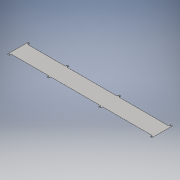
# Autodesk Inventor part: Baseplate
Saved by Autodesk Inventor 2016 (Build 200138000, 138)
## iProperties
Created: 2017-06-28
Part Number: Baseplate
Material: Generic
Document SubType Name: Modeling
Designer: Roeder
Density: 1 g/cm^3
Appearance: Default
Author: Roeder
Autodesk Inventor part; units mm, degrees
ref_plane "YZ Plane" through (0, 0, 0) normal (1, 0, 0) x (0, 1, 0)
ref_plane "XZ Plane" through (0, 0, 0) normal (0, 1, 0) x (-1, 0, 0)
ref_plane "XY Plane" through (0, 0, 0) normal (0, 0, 1) x (1, 0, 0)
sketch "Sketch1" plane through (0, 0, 0) normal (0, 0, 1) x (1, 0, 0)
  line L0 (-836.3865, 0) -> (4049.6135, 0) projected
  line L1 (0, -497.7012) -> (0, 202.2988) projected
  line L2 (-93.3865, 52.2988) -> (3306.6135, 52.2988)
  line L3 (3306.6135, 52.2988) -> (3306.6135, -347.7012)
  line L4 (3306.6135, -347.7012) -> (-93.3865, -347.7012)
  line L5 (-93.3865, -347.7012) -> (-93.3865, 52.2988)
  line L6 (-93.3865, 52.2988) -> (-93.3865, 102.2988)
  line L7 (-93.3865, 102.2988) -> (-138.3865, 102.2988)
  line L8 (-138.3865, 102.2988) -> (-138.3865, -397.7012)
  line L9 (-138.3865, -397.7012) -> (-93.3865, -397.7012)
  line L10 (-93.3865, -397.7012) -> (-93.3865, -347.7012)
  line L11 (3306.6135, -347.7012) -> (3306.6135, -397.7012)
  line L12 (3306.6135, -397.7012) -> (3351.6135, -397.7012)
  line L13 (3351.6135, -397.7012) -> (3351.6135, 102.2988)
  line L14 (3351.6135, 102.2988) -> (3306.6135, 102.2988)
  line L15 (3306.6135, 102.2988) -> (3306.6135, 52.2988)
  line L16 (811.6135, 52.2988) -> (811.6135, 97.2988)
  line L17 (811.6135, 97.2988) -> (856.6135, 97.2988)
  line L18 (856.6135, 97.2988) -> (856.6135, 52.2988)
  line L19 (811.6135, 52.2988) -> (811.6135, -347.7012)
  line L20 (811.6135, -397.7012) -> (856.6135, -397.7012)
  line L21 (856.6135, -397.7012) -> (856.6135, -347.7012)
  line L22 (856.6135, 52.2988) -> (856.6135, -347.7012)
  line L23 (811.6135, -347.7012) -> (811.6135, -397.7012)
  line L24 (2061.6135, 52.2988) -> (2061.6135, 102.2988)
  line L25 (2061.6135, 102.2988) -> (2106.6135, 102.2988)
  line L26 (2106.6135, 102.2988) -> (2106.6135, 52.2988)
  line L27 (2106.6135, -347.7012) -> (2106.6135, 52.2988)
  line L28 (2106.6135, -347.7012) -> (2106.6135, -397.7012)
  line L29 (2106.6135, -397.7012) -> (2061.6135, -397.7012)
  line L30 (2061.6135, -397.7012) -> (2061.6135, -347.7012)
  line L31 (2061.6135, -347.7012) -> (2061.6135, 52.2988)
  dimension "d2" = 3400
  dimension "d3" = 400
  dimension "d4" = 50
  dimension "d5" = 45
  dimension "d6" = 500
  dimension "d7" = 50
  dimension "d8" = 45
  dimension "d9" = 45
  dimension "d10" = 905
  dimension "d11" = 45
  dimension "d12" = 45
  dimension "d13" = 1200
  constraints: 60 end point, 17 perpendicular, 15 point on line, 5 vertical, 3 parallel, 2 horizontal, 1 collinear
  measures "d2" distance of L3.end L4.end
  measures "d3" distance of L2.end L3.end
  measures "d4" distance of L2.start L6.end
  measures "d5" distance of L6.end L7.end
  measures "d6" distance of L7.end L8.end
  measures "d7" distance of L3.end L11.end
  measures "d8" distance of L11.end L12.end
  measures "d9" distance of L16.end L17.end
  measures "d10" distance between parallel lines of L16 L6
  measures "d11" distance of L24.end L25.end
  measures "d12" distance between parallel lines of L17 L2
  measures "d13" distance between parallel lines of L15 L26
extrude "Extrusion1" add sketch "Sketch1" along normal blind 2
sketch "Sketch2" plane through (0, 0, 2) normal (0, 0, 1) x (1, 0, 0)
  line L0 (-123.3865, 82.2988) -> (-108.3865, 82.2988)
  line L1 (-123.3865, 72.2988) -> (-108.3865, 72.2988)
  line L2 (-195.8041, 77.2988) -> (3412.5269, 77.2988) construction
  line L3 (811.6135, 52.2988) -> (-93.3865, 52.2988) construction
  line L4 (-93.3865, 102.2988) -> (-138.3865, 102.2988) construction
  line L5 (-115.8865, 102.2988) -> (-115.8865, -482.0806) construction
  arc A0 (-123.3865, 82.2988) -> (-123.3865, 72.2988) centre (-123.3865, 77.2988) ccw
  arc A1 (-108.3865, 72.2988) -> (-108.3865, 82.2988) centre (-108.3865, 77.2988) ccw
  line L6 (-166.4854, -372.7012) -> (3412.5269, -372.7012) construction
  line L7 (3351.6135, 102.2988) -> (3306.6135, 102.2988) construction
  line L8 (3329.1135, 102.2988) -> (3329.1135, -396.0757) construction
  line L9 (2106.6135, 102.2988) -> (2061.6135, 102.2988) construction
  line L10 (2084.1135, 102.2988) -> (2084.1135, -396.0757) construction
  line L11 (-93.3865, -347.7012) -> (811.6135, -347.7012) construction
  line L12 (-138.3865, 102.2988) -> (-138.3865, -397.7012) construction
  line L13 (-138.3865, -147.7012) -> (3351.6135, -147.7012) construction
  line L14 (3351.6135, -397.7012) -> (3351.6135, 102.2988) construction
  line L15 (856.6135, 97.2988) -> (811.6135, 97.2988) construction
  line L16 (834.1135, 97.2988) -> (834.1135, -397.7012) construction
  line L17 (-123.3865, -367.7012) -> (-108.3865, -367.7012)
  line L18 (-123.3865, -377.7012) -> (-108.3865, -377.7012)
  arc A2 (-123.3865, -367.7012) -> (-123.3865, -377.7012) centre (-123.3865, -372.7012) ccw
  arc A3 (-108.3865, -377.7012) -> (-108.3865, -367.7012) centre (-108.3865, -372.7012) ccw
  line L19 (826.6135, 82.2988) -> (841.6135, 82.2988)
  line L20 (826.6135, 72.2988) -> (841.6135, 72.2988)
  arc A4 (826.6135, 82.2988) -> (826.6135, 72.2988) centre (826.6135, 77.2988) ccw
  arc A5 (841.6135, 72.2988) -> (841.6135, 82.2988) centre (841.6135, 77.2988) ccw
  line L21 (826.6135, -367.7012) -> (841.6135, -367.7012)
  line L22 (826.6135, -377.7012) -> (841.6135, -377.7012)
  arc A6 (826.6135, -367.7012) -> (826.6135, -377.7012) centre (826.6135, -372.7012) ccw
  arc A7 (841.6135, -377.7012) -> (841.6135, -367.7012) centre (841.6135, -372.7012) ccw
  line L23 (2076.6135, 82.2988) -> (2091.6135, 82.2988)
  line L24 (2076.6135, 72.2988) -> (2091.6135, 72.2988)
  arc A8 (2076.6135, 82.2988) -> (2076.6135, 72.2988) centre (2076.6135, 77.2988) ccw
  arc A9 (2091.6135, 72.2988) -> (2091.6135, 82.2988) centre (2091.6135, 77.2988) ccw
  line L25 (2076.6135, -367.7012) -> (2091.6135, -367.7012)
  line L26 (2076.6135, -377.7012) -> (2091.6135, -377.7012)
  arc A10 (2076.6135, -367.7012) -> (2076.6135, -377.7012) centre (2076.6135, -372.7012) ccw
  arc A11 (2091.6135, -377.7012) -> (2091.6135, -367.7012) centre (2091.6135, -372.7012) ccw
  line L27 (3321.6135, 82.2988) -> (3336.6135, 82.2988)
  line L28 (3321.6135, 72.2988) -> (3336.6135, 72.2988)
  arc A12 (3321.6135, 82.2988) -> (3321.6135, 72.2988) centre (3321.6135, 77.2988) ccw
  arc A13 (3336.6135, 72.2988) -> (3336.6135, 82.2988) centre (3336.6135, 77.2988) ccw
  line L29 (3321.6135, -367.7012) -> (3336.6135, -367.7012)
  line L30 (3321.6135, -377.7012) -> (3336.6135, -377.7012)
  arc A14 (3321.6135, -367.7012) -> (3321.6135, -377.7012) centre (3321.6135, -372.7012) ccw
  arc A15 (3336.6135, -377.7012) -> (3336.6135, -367.7012) centre (3336.6135, -372.7012) ccw
  point P0 (0, 0)
  point P1 (-115.8865, 77.2988)
  point P2 (-115.8865, -372.7012)
  point P3 (834.1135, -372.7012)
  point P4 (834.1135, 77.2988)
  point P5 (2084.1135, 77.2988)
  point P6 (2084.1135, -372.7012)
  point P7 (3329.1135, 77.2988)
  point P8 (3329.1135, -372.7012)
  point P9 (-115.8865, -372.7012)
  point P10 (834.1135, 77.2988)
  point P11 (834.1135, -372.7012)
  point P12 (2084.1135, 77.2988)
  point P13 (2084.1135, -372.7012)
  point P14 (3329.1135, 77.2988)
  point P15 (3329.1135, -372.7012)
  dimension "d16" = 15
  dimension "d18" = 15
  dimension "d20" = 0
  dimension "d21" = 0
  dimension "d52" = 25
  dimension "d53" = 25
  dimension "d54" = 15
  dimension "d55" = 15
  dimension "d56" = 0
  dimension "d57" = 0
  dimension "d58" = 15
  dimension "d59" = 15
  dimension "d60" = 0
  dimension "d61" = 0
  dimension "d62" = 15
  dimension "d63" = 15
  dimension "d64" = 0
  dimension "d65" = 0
  dimension "d66" = 15
  dimension "d67" = 15
  dimension "d68" = 0
  dimension "d69" = 0
  dimension "d70" = 15
  dimension "d71" = 15
  dimension "d72" = 0
  dimension "d73" = 0
  dimension "d74" = 15
  dimension "d75" = 15
  dimension "d76" = 0
  dimension "d77" = 0
  dimension "d78" = 15
  dimension "d79" = 15
  dimension "d80" = 0
  dimension "d81" = 0
  constraints: 48 point on line, 46 end point, 32 point on circle, 18 horizontal, 16 centre point, 16 tangent, 6 midpoint, 3 symmetric about line, 3 vertical, 1 perpendicular, 1 other
  measures "d16" distance of L0.start L0.end
  measures "d18" distance of L1.start L1.end
  measures "d20" distance of L0.start A0.start
  measures "d21" distance of L0.end A1.end
  measures "d52" distance between parallel lines of L2 L3
  measures "d53" distance between parallel lines of L6 L11
  measures "d54" distance of L17.start L17.end
  measures "d55" distance of L18.start L18.end
  measures "d56" distance of L17.start A2.start
  measures "d57" distance of L17.end A3.end
  measures "d58" distance of L19.start L19.end
  measures "d59" distance of L20.start L20.end
  measures "d60" distance of L19.start A4.start
  measures "d61" distance of L19.end A5.end
  measures "d62" distance of L21.start L21.end
  measures "d63" distance of L22.start L22.end
  measures "d64" distance of L21.start A6.start
  measures "d65" distance of L21.end A7.end
  measures "d66" distance of L23.start L23.end
  measures "d67" distance of L24.start L24.end
  measures "d68" distance of L23.start A8.start
  measures "d69" distance of L23.end A9.end
  measures "d70" distance of L25.start L25.end
  measures "d71" distance of L26.start L26.end
  measures "d72" distance of L25.start A10.start
  measures "d73" distance of L25.end A11.end
  measures "d74" distance of L27.start L27.end
  measures "d75" distance of L28.start L28.end
  measures "d76" distance of L27.start A12.start
  measures "d77" distance of L27.end A13.end
  measures "d78" distance of L29.start L29.end
  measures "d79" distance of L30.start L30.end
  measures "d80" distance of L29.start A14.start
  measures "d81" distance of L29.end A15.end
extrude "Extrusion2" cut sketch "Sketch2" against normal blind 20
body "Solid1"
